Autodesk Inventor part; units mm, degrees
(part 2 of 2)
sketch "Sketch27" plane through (0, 0, 6.35) normal (0, 0, 1) x (1, 0, 0)
  line L0 (-73.9957, 172.4284) -> (-73.9957, 166.0784) projected
  line L1 (-73.9957, 166.0784) -> (-124.7957, 166.0784) projected
  line L2 (-124.7957, 166.0784) -> (-124.7957, 172.4284) projected
  line L3 (-143.8457, 172.4284) -> (-124.7957, 172.4284) projected
  line L4 (351.4543, -640.3716) -> (351.4543, -716.5716) projected
  line L5 (351.4543, -640.3716) -> (345.1043, -640.3716) projected
  line L6 (345.1043, -640.3716) -> (345.1043, -589.5716) projected
  line L7 (345.1043, -589.5716) -> (351.4543, -589.5716) projected
  line L8 (351.4543, -538.7716) -> (351.4543, -589.5716) projected
  line L9 (351.4543, -538.7716) -> (345.1043, -538.7716) projected
  line L10 (345.1043, -538.7716) -> (345.1043, -487.9716) projected
  line L11 (345.1043, -487.9716) -> (351.4543, -487.9716) projected
  line L12 (351.4543, -437.1716) -> (351.4543, -487.9716) projected
  line L13 (351.4543, -437.1716) -> (345.1043, -437.1716) projected
  line L14 (345.1043, -437.1716) -> (345.1043, -386.3716) projected
  line L15 (345.1043, -386.3716) -> (351.4543, -386.3716) projected
  line L16 (351.4543, -335.5716) -> (351.4543, -386.3716) projected
  line L17 (351.4543, -335.5716) -> (345.1043, -335.5716) projected
  line L18 (345.1043, -335.5716) -> (345.1043, -284.7716) projected
  line L19 (345.1043, -284.7716) -> (351.4543, -284.7716) projected
  line L20 (351.4543, -233.9716) -> (351.4543, -284.7716) projected
  line L21 (351.4543, -233.9716) -> (345.1043, -233.9716) projected
  line L22 (345.1043, -233.9716) -> (345.1043, -183.1716) projected
  line L23 (345.1043, -183.1716) -> (351.4543, -183.1716) projected
  line L24 (351.4543, -132.3716) -> (351.4543, -183.1716) projected
  line L25 (351.4543, -132.3716) -> (345.1043, -132.3716) projected
  line L26 (345.1043, -132.3716) -> (345.1043, -81.5716) projected
  line L27 (345.1043, -81.5716) -> (351.4543, -81.5716) projected
  line L28 (351.4543, -30.7716) -> (351.4543, -81.5716) projected
  line L29 (351.4543, -30.7716) -> (345.1043, -30.7716) projected
  line L30 (345.1043, -30.7716) -> (345.1043, 20.0284) projected
  line L31 (345.1043, 20.0284) -> (351.4543, 20.0284) projected
  line L32 (351.4543, 70.8284) -> (351.4543, 20.0284) projected
  line L33 (351.4543, 70.8284) -> (345.1043, 70.8284) projected
  line L34 (345.1043, 70.8284) -> (345.1043, 121.6284) projected
  line L35 (345.1043, 121.6284) -> (351.4543, 121.6284) projected
  line L36 (351.4543, 172.4284) -> (351.4543, 121.6284) projected
  line L37 (332.4043, 172.4284) -> (351.4543, 172.4284) projected
  line L38 (332.4043, 172.4284) -> (332.4043, 166.0784) projected
  line L39 (332.4043, 166.0784) -> (281.6043, 166.0784) projected
  line L40 (281.6043, 166.0784) -> (281.6043, 172.4284) projected
  line L41 (230.8043, 172.4284) -> (281.6043, 172.4284) projected
  line L42 (230.8043, 172.4284) -> (230.8043, 166.0784) projected
  line L43 (230.8043, 166.0784) -> (180.0043, 166.0784) projected
  line L44 (180.0043, 166.0784) -> (180.0043, 172.4284) projected
  line L45 (129.2043, 172.4284) -> (180.0043, 172.4284) projected
  line L46 (129.2043, 172.4284) -> (129.2043, 166.0784) projected
  line L47 (129.2043, 166.0784) -> (78.4043, 166.0784) projected
  line L48 (78.4043, 166.0784) -> (78.4043, 172.4284) projected
  line L49 (27.6043, 172.4284) -> (78.4043, 172.4284) projected
  line L50 (27.6043, 172.4284) -> (27.6043, 166.0784) projected
  line L51 (27.6043, 166.0784) -> (-23.1957, 166.0784) projected
  line L52 (-23.1957, 166.0784) -> (-23.1957, 172.4284) projected
  line L53 (-73.9957, 172.4284) -> (-23.1957, 172.4284) projected
  line L54 (-143.8457, 172.4284) -> (351.4543, 172.4284)
  line L55 (351.4543, 172.4284) -> (351.4543, -716.5716)
  line L56 (351.4543, -716.5716) -> (-143.8457, -716.5716)
  line L57 (-143.8457, -716.5716) -> (-143.8457, 172.4284)
  line L58 (-113.7837, 147.0284) -> (316.8841, 147.0284)
  line L59 (316.8841, 147.0284) -> (316.8841, -678.4716)
  line L60 (316.8841, -678.4716) -> (-113.7837, -678.4716)
  line L61 (-113.7837, -678.4716) -> (-113.7837, 147.0284)
  point P0 (0, 0)
  constraints: 16 end point, 4 parallel, 2 horizontal, 2 perpendicular
extrude "Extrusion27" add sketch "Sketch27" against normal blind 6.35 contours L0 L1 L2 L54 | L54 L50 L51 L52 | L54 L46 L47 L48 | L54 L42 L43 L44 | L5 L6 L7 L55 | L54 L38 L39 L40 | L9 L10 L11 L55 | L13 L14 L15 L55 | L55 L33 L34 L35 | L17 L18 L19 L55 | L55 L29 L30 L31 | L21 L22 L23 L55 | L55 L25 L26 L27
sketch "Sketch28" plane through (0, 0, 6.35) normal (0, 0, 1) x (1, 0, 0)
  line L0 (-143.8457, 172.4284) -> (351.4543, 172.4284) projected
  line L1 (-143.8457, 121.6284) -> (-143.8457, 172.4284) projected
  line L2 (-143.8457, 121.6284) -> (-137.4957, 121.6284) projected
  line L3 (-137.4957, 121.6284) -> (-137.4957, 70.8284) projected
  line L4 (-137.4957, 70.8284) -> (-143.8457, 70.8284) projected
  line L5 (-143.8457, 20.0284) -> (-143.8457, 70.8284) projected
  line L6 (-143.8457, 20.0284) -> (-137.4957, 20.0284) projected
  line L7 (-137.4957, 20.0284) -> (-137.4957, -30.7716) projected
  line L8 (-137.4957, -30.7716) -> (-143.8457, -30.7716) projected
  line L9 (-143.8457, -81.5716) -> (-143.8457, -30.7716) projected
  line L10 (-143.8457, -81.5716) -> (-137.4957, -81.5716) projected
  line L11 (-137.4957, -81.5716) -> (-137.4957, -132.3716) projected
  line L12 (-137.4957, -132.3716) -> (-143.8457, -132.3716) projected
  line L13 (-143.8457, -183.1716) -> (-143.8457, -132.3716) projected
  line L14 (-143.8457, -183.1716) -> (-137.4957, -183.1716) projected
  line L15 (-137.4957, -183.1716) -> (-137.4957, -233.9716) projected
  line L16 (-137.4957, -233.9716) -> (-143.8457, -233.9716) projected
  line L17 (-143.8457, -284.7716) -> (-143.8457, -233.9716) projected
  line L18 (-143.8457, -284.7716) -> (-137.4957, -284.7716) projected
  line L19 (-137.4957, -284.7716) -> (-137.4957, -335.5716) projected
  line L20 (-137.4957, -335.5716) -> (-143.8457, -335.5716) projected
  line L21 (-143.8457, -386.3716) -> (-143.8457, -335.5716) projected
  line L22 (-143.8457, -386.3716) -> (-137.4957, -386.3716) projected
  line L23 (-137.4957, -386.3716) -> (-137.4957, -437.1716) projected
  line L24 (-137.4957, -437.1716) -> (-143.8457, -437.1716) projected
  line L25 (-143.8457, -487.9716) -> (-143.8457, -437.1716) projected
  line L26 (-143.8457, -487.9716) -> (-137.4957, -487.9716) projected
  line L27 (-137.4957, -487.9716) -> (-137.4957, -538.7716) projected
  line L28 (-137.4957, -538.7716) -> (-143.8457, -538.7716) projected
  line L29 (-143.8457, -589.5716) -> (-143.8457, -538.7716) projected
  line L30 (-143.8457, -589.5716) -> (-137.4957, -589.5716) projected
  line L31 (-137.4957, -589.5716) -> (-137.4957, -640.3716) projected
  line L32 (-137.4957, -640.3716) -> (-143.8457, -640.3716) projected
  line L33 (-143.8457, -716.5716) -> (-143.8457, -640.3716) projected
  line L34 (-124.7957, -716.5716) -> (-143.8457, -716.5716) projected
  line L35 (-124.7957, -716.5716) -> (-124.7957, -710.2216) projected
  line L36 (-124.7957, -710.2216) -> (-73.9957, -710.2216) projected
  line L37 (-73.9957, -710.2216) -> (-73.9957, -716.5716) projected
  line L38 (-23.1957, -716.5716) -> (-73.9957, -716.5716) projected
  line L39 (-23.1957, -716.5716) -> (-23.1957, -710.2216) projected
  line L40 (-23.1957, -710.2216) -> (27.6043, -710.2216) projected
  line L41 (27.6043, -710.2216) -> (27.6043, -716.5716) projected
  line L42 (78.4043, -716.5716) -> (27.6043, -716.5716) projected
  line L43 (78.4043, -716.5716) -> (78.4043, -710.2216) projected
  line L44 (78.4043, -710.2216) -> (129.2043, -710.2216) projected
  line L45 (129.2043, -710.2216) -> (129.2043, -716.5716) projected
  line L46 (180.0043, -716.5716) -> (129.2043, -716.5716) projected
  line L47 (180.0043, -716.5716) -> (180.0043, -710.2216) projected
  line L48 (180.0043, -710.2216) -> (230.8043, -710.2216) projected
  line L49 (230.8043, -710.2216) -> (230.8043, -716.5716) projected
  line L50 (281.6043, -716.5716) -> (230.8043, -716.5716) projected
  line L51 (281.6043, -716.5716) -> (281.6043, -710.2216) projected
  line L52 (281.6043, -710.2216) -> (332.4043, -710.2216) projected
  line L53 (332.4043, -710.2216) -> (332.4043, -716.5716) projected
  line L54 (351.4543, -716.5716) -> (332.4043, -716.5716) projected
  line L55 (351.4543, 172.4284) -> (351.4543, -716.5716) projected
  line L56 (129.2043, -481.6216) -> (78.4043, -481.6216) projected
  line L57 (-143.8457, 121.6284) -> (-143.8457, -640.3716)
  point P0 (0, 0)
  constraints: 2 end point, 1 perpendicular
extrude "Extrusion28" add sketch "Sketch28" against normal blind 6.35 contours L2 L3 L4 L57 | L6 L7 L8 L57 | L10 L11 L12 L57 | L14 L15 L16 L57 | L18 L19 L20 L57 | L22 L23 L24 L57 | L26 L27 L28 L57 | L30 L31 L32 L57
sketch "Sketch29" plane through (0, 0, 6.35) normal (0, 0, 1) x (1, 0, 0)
  line L0 (-143.8457, 172.4284) -> (351.4543, 172.4284) projected
  line L1 (-143.8457, -716.5716) -> (-143.8457, 172.4284) projected
  line L2 (-124.7957, -716.5716) -> (-143.8457, -716.5716) projected
  line L3 (-124.7957, -716.5716) -> (-124.7957, -710.2216) projected
  line L4 (-124.7957, -710.2216) -> (-73.9957, -710.2216) projected
  line L5 (-73.9957, -710.2216) -> (-73.9957, -716.5716) projected
  line L6 (-23.1957, -716.5716) -> (-73.9957, -716.5716) projected
  line L7 (-23.1957, -716.5716) -> (-23.1957, -710.2216) projected
  line L8 (-23.1957, -710.2216) -> (27.6043, -710.2216) projected
  line L9 (27.6043, -710.2216) -> (27.6043, -716.5716) projected
  line L10 (78.4043, -716.5716) -> (27.6043, -716.5716) projected
  line L11 (78.4043, -716.5716) -> (78.4043, -710.2216) projected
  line L12 (78.4043, -710.2216) -> (129.2043, -710.2216) projected
  line L13 (129.2043, -710.2216) -> (129.2043, -716.5716) projected
  line L14 (180.0043, -716.5716) -> (129.2043, -716.5716) projected
  line L15 (180.0043, -716.5716) -> (180.0043, -710.2216) projected
  line L16 (180.0043, -710.2216) -> (230.8043, -710.2216) projected
  line L17 (230.8043, -710.2216) -> (230.8043, -716.5716) projected
  line L18 (281.6043, -716.5716) -> (230.8043, -716.5716) projected
  line L19 (281.6043, -716.5716) -> (281.6043, -710.2216) projected
  line L20 (281.6043, -710.2216) -> (332.4043, -710.2216) projected
  line L21 (332.4043, -710.2216) -> (332.4043, -716.5716) projected
  line L22 (351.4543, -716.5716) -> (332.4043, -716.5716) projected
  line L23 (351.4543, 172.4284) -> (351.4543, -716.5716) projected
  line L24 (129.2043, -481.6216) -> (78.4043, -481.6216) projected
  line L25 (-124.7957, -716.5716) -> (332.4043, -716.5716)
  point P0 (0, 0)
  constraints: 2 end point, 1 parallel
extrude "Extrusion29" add sketch "Sketch29" against normal blind 6.35 contours L3 L4 L5 L25 | L25 L19 L20 L21 | L7 L8 L9 L25 | L25 L15 L16 L17 | L11 L12 L13 L25
sketch "Sketch30" plane through (0, 0, 0) normal (0, 0, -1) x (-1, 0, 0)
  circle A0 centre (-103.8043, -212.0514) radius 2.3495 projected
  line L0 (143.8457, 172.4284) -> (-351.4543, 172.4284) projected
  line L1 (-351.4543, 172.4284) -> (-351.4543, -716.5716) projected
  line L2 (143.8457, -716.5716) -> (143.8457, 172.4284) projected
  line L3 (-351.4543, -716.5716) -> (143.8457, -716.5716)
  line L4 (143.8457, -716.5716) -> (143.8457, -399.097)
  line L5 (143.8457, -399.097) -> (-351.4543, -399.097)
  line L6 (-351.4543, -399.097) -> (-351.4543, -716.5716)
  point P0 (0, 0)
  dimension "d163" = 317.4746
  constraints: 8 end point, 2 parallel, 1 horizontal, 1 perpendicular, 1 point on line
  measures "d163" distance of L4.end L3.end
extrude "Extrusion30" cut sketch "Sketch30" against normal blind 25.4 contours L2 L5 L1 L0
sketch "Sketch31" plane through (0, 0, 0) normal (0, 0, -1) x (-1, 0, 0)
  line L0 (143.8457, -399.097) -> (-351.4543, -399.097) projected
  line L1 (-103.8043, -399.097) -> (-141.9043, -399.097)
  line L2 (-141.9043, -399.097) -> (-65.7043, -399.097)
  line L3 (-65.7043, -399.097) -> (-65.7043, -183.197)
  line L4 (-65.7043, -183.197) -> (-141.9043, -183.197)
  line L5 (-141.9043, -183.197) -> (-141.9043, -399.097)
  point P0 (0, 0)
  dimension "d166" = 38.1
  dimension "d167" = 76.2
  dimension "d168" = 215.9
  constraints: 10 end point, 2 parallel, 1 horizontal, 1 midpoint, 1 perpendicular, 1 point on line
  measures "d166" distance of L1.start L1.end
  measures "d167" distance of L4.end L3.end
  measures "d168" distance of L3.end L2.end
extrude "Extrusion31" add sketch "Sketch31" against normal blind 6.35
sketch "Sketch32" plane through (0, 0, 0) normal (0, 0, -1) x (-1, 0, 0)
  circle A0 centre (-103.8043, -430.3009) radius 2.3495 projected
  line L0 (-281.6043, -468.9216) -> (-230.8043, -468.9216) projected
  line L1 (-103.8043, -430.3009) -> (-103.8043, -212.0387)
  circle A1 centre (-103.8043, -212.0387) radius 2.3495
  point P0 (0, 0)
  dimension "d171" = 218.2622
  constraints: 2 end point, 1 centre point, 1 coincident, 1 perpendicular
  measures "d171" distance of L1.start L1.end
extrude "Extrusion32" cut sketch "Sketch32" against normal blind 6.35 contours A1
sketch "Sketch33" plane through (0, 0, 0) normal (0, 0, -1) x (-1, 0, 0)
  line L0 (143.8457, -716.5716) -> (143.8457, -399.097) projected
  line L1 (-351.4543, -399.097) -> (-141.9043, -399.097)
  line L2 (-141.9043, -399.097) -> (-141.9043, -405.447)
  line L3 (-141.9043, -405.447) -> (-351.4543, -405.447)
  line L4 (-351.4543, -405.447) -> (-351.4543, -399.097)
  line L5 (-65.7043, -399.097) -> (143.8457, -399.097)
  line L6 (143.8457, -399.097) -> (143.8457, -405.447)
  line L7 (143.8457, -405.447) -> (-65.7043, -405.447)
  line L8 (-65.7043, -405.447) -> (-65.7043, -399.097)
  point P0 (0, 0)
  dimension "d174" = 6.35
  constraints: 16 end point, 4 parallel, 2 horizontal, 2 perpendicular, 1 point on line
  measures "d174" distance of L1.end L2.end
extrude "Extrusion33" cut sketch "Sketch33" against normal blind 25.4
sketch "Sketch34" plane through (0, 0, 0) normal (0, 0, -1) x (-1, 0, 0)
  line L0 (-351.4543, -405.447) -> (-262.5543, -405.447)
  line L1 (-262.5543, -405.447) -> (-262.5543, -411.797)
  line L2 (-262.5543, -411.797) -> (-351.4543, -411.797)
  line L3 (-351.4543, -411.797) -> (-351.4543, -405.447)
  line L4 (143.8457, -405.447) -> (54.9457, -405.447)
  line L5 (54.9457, -405.447) -> (54.9457, -411.797)
  line L6 (54.9457, -411.797) -> (143.8457, -411.797)
  line L7 (143.8457, -411.797) -> (143.8457, -405.447)
  point P0 (0, 0)
  dimension "d177" = 88.9
  dimension "d178" = 6.35
  dimension "d179" = 88.9
  dimension "d180" = 6.35
  constraints: 16 end point, 4 parallel, 2 horizontal, 2 perpendicular
  measures "d177" distance of L1.end L2.end
  measures "d178" distance of L0.end L1.end
  measures "d179" distance of L6.end L5.end
  measures "d180" distance of L5.end L4.end
extrude "Extrusion34" cut sketch "Sketch34" against normal blind 25.4
sketch "Sketch35" plane through (0, 0, 0) normal (0, 0, -1) x (-1, 0, 0)
  line L0 (-230.8043, -468.9216) -> (-230.8043, -481.6216) projected
  line L1 (-230.8043, -481.6216) -> (-281.6043, -481.6216) projected
  line L2 (-281.6043, -481.6216) -> (-281.6043, -468.9216) projected
  line L3 (-281.6043, -468.9216) -> (-230.8043, -468.9216) projected
  line L4 (-78.4043, -468.9216) -> (-78.4043, -481.6216) projected
  line L5 (-78.4043, -481.6216) -> (-129.2043, -481.6216) projected
  line L6 (-129.2043, -481.6216) -> (-129.2043, -468.9216) projected
  line L7 (-129.2043, -468.9216) -> (-78.4043, -468.9216) projected
  line L8 (73.9957, -468.9216) -> (73.9957, -481.6216) projected
  line L9 (73.9957, -481.6216) -> (23.1957, -481.6216) projected
  line L10 (23.1957, -481.6216) -> (23.1957, -468.9216) projected
  line L11 (23.1957, -468.9216) -> (73.9957, -468.9216) projected
  point P0 (0, 0)
extrude "Extrusion35" add sketch "Sketch35" against normal blind 6.35
sketch "Sketch36" plane through (0, 0, 6.35) normal (0, 0, 1) x (1, 0, 0)
  line L0 (262.5543, -411.797) -> (351.4543, -411.797)
  line L1 (351.4543, -411.797) -> (351.4543, -405.447)
  line L2 (351.4543, -405.447) -> (262.5543, -405.447)
  line L3 (262.5543, -405.447) -> (262.5543, -411.797)
  line L4 (-54.9457, -411.797) -> (-143.8457, -411.797)
  line L5 (-143.8457, -411.797) -> (-143.8457, -405.447)
  line L6 (-143.8457, -405.447) -> (-54.9457, -405.447)
  line L7 (-54.9457, -405.447) -> (-54.9457, -411.797)
  point P0 (0, 0)
  constraints: 16 end point, 4 parallel, 2 horizontal, 2 perpendicular
extrude "Extrusion36" add sketch "Sketch36" against normal blind 6.35
body "Solid1"
